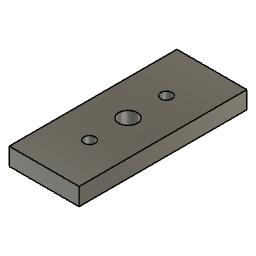
후방 덮개 브라켓2 (Autodesk Fusion 360 design; units mm, degrees)
Autodesk Fusion 360 part; units mm, degrees
sketch "스케치1" plane through (0, 0, 0) normal (0, 0, 1) x (1, 0, 0)
  line L0 (10, 24) -> (-10, 24)
  line L1 (-10, 24) -> (-10, -24)
  line L2 (-10, -24) -> (10, -24)
  line L3 (10, -24) -> (10, 24)
  line L4 (10, 24) -> (-10, -24) construction
  line L5 (-10, 24) -> (10, -24) construction
  line L6 (0, 0) -> (0, 11)
  circle A0 centre (0, 11) radius 1.6
  line L7 (0, 0) -> (0, -11)
  circle A1 centre (0, -11) radius 1.6
  circle A2 centre (0, 0) radius 2.65
  dimension "d1" = 20
  dimension "d2" = 48
  dimension "d3" = 11
  dimension "d4" = 3.2
  dimension "d5" = 11
  dimension "d6" = 3.2
  dimension "d7" = 5.3
  constraint horizontal L0
  constraint perpendicular L0 L1
  constraint parallel L0 L2
  constraint parallel L1 L3
  constraint coincident L4 L6.start
  constraint coincident L5 L6.start
  constraint coincident L6.start L7.start
  constraint perpendicular L0 L6
  constraint coincident L6.end A0.centre
  constraint parallel L6 L7
  constraint coincident L7.end A1.centre
  measures "d1" distance of L1.end L2.end
  measures "d2" distance of L0.end L1.end
  measures "d3" distance of L6.start L6.end
  measures "d4" diameter of A0
  measures "d5" distance of L6.start L7.end
  measures "d6" diameter of A1
  measures "d7" diameter of A2
extrude "돌출1" add sketch "스케치1" along normal blind 5
extrude "돌출2" add sketch "스케치1" along normal blind 2.8 contours A0 | A1
